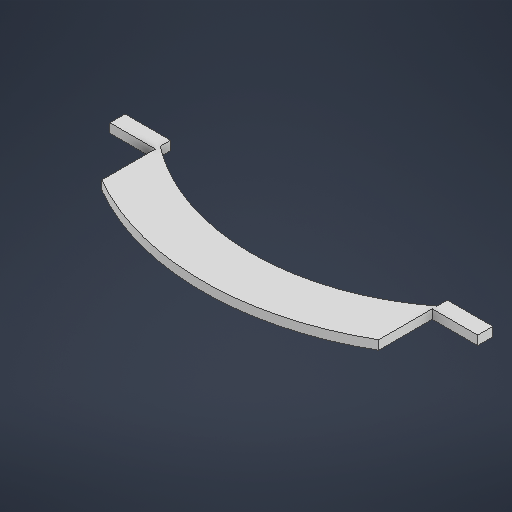
# Autodesk Inventor part: Pieza Contramolde
Saved by Autodesk Inventor 2026.2 (Build 302298000, 298)
## iProperties
Created: 2026-02-26
Part Number: Pieza Contramolde
Material: Generic
Document SubType Name: Modeling
Designer: 06aar
Density: 1 g/cm^3
Appearance: Default
Author: 06aar
Autodesk Inventor part; units mm, degrees
ref_plane "YZ Plane" through (0, 0, 0) normal (1, 0, 0) x (0, 1, 0)
ref_plane "XZ Plane" through (0, 0, 0) normal (0, 1, 0) x (-1, 0, 0)
ref_plane "XY Plane" through (0, 0, 0) normal (0, 0, 1) x (1, 0, 0)
sketch "Sketch1" plane through (0, 0, 0) normal (0, 1, 0) x (-1, 0, 0)
  circle A0 centre (0, 0) radius 75
  line L0 (0, 0) -> (45.6571, 59.5015)
  line L1 (0, 0) -> (-45.6571, 59.5015)
  line L2 (0, 0) -> (0, 75)
  circle A1 centre (0, 0) radius 72.3
  circle A2 centre (0, 0) radius 91
  line L3 (45.6571, 59.5015) -> (45.6571, 56.06)
  line L4 (45.6571, 56.06) -> (60.6571, 56.06)
  line L5 (45.6571, 59.5015) -> (45.6571, 78.7174)
  line L6 (60.6571, 56.06) -> (60.6571, 61.06)
  line L7 (60.6571, 61.06) -> (45.6571, 61.06)
  line L8 (-45.6571, 59.5015) -> (-45.6571, 56.06)
  line L9 (-45.6571, 56.06) -> (-60.6571, 56.06)
  line L10 (-45.6571, 59.5015) -> (-45.6571, 78.7174)
  line L11 (-60.6571, 56.06) -> (-60.6571, 61.06)
  line L12 (-60.6571, 61.06) -> (-45.6571, 61.06)
  point P0 (44.0135, 57.3594)
  point P1 (-44.0135, 57.3594)
  dimension "d0" = 150
  dimension "d1" = 37.5
  dimension "d2" = 37.5
  dimension "d3" = 2.7
  dimension "d9" = 16
  dimension "d21" = 15
  dimension "d22" = 5
  constraints: 26 end point, 8 point on circle, 5 vertical, 4 point on line, 4 symmetric about line, 3 centre point, 3 coincident, 1 concentric, 1 horizontal, 1 perpendicular
  measures "d0" diameter of A0
  measures "d1" angle of L1 L2
  measures "d2" angle of L2 L0
  measures "d3" radial gap between concentric circles of A0 A1
  measures "d9" radial gap between concentric circles of A2 A0
  measures "d21" distance of L3.end L4.end
  measures "d22" distance between parallel lines of L4 L7
extrude "Extrusion1" add sketch "Sketch1" along normal blind 3 contours L5 L7 L6 L4 A0 | A0 L4 L3 | A0 L10 A2 L5 | L8 L9 A0 | A0 L9 L11 L12 L10
body "Solid1"
